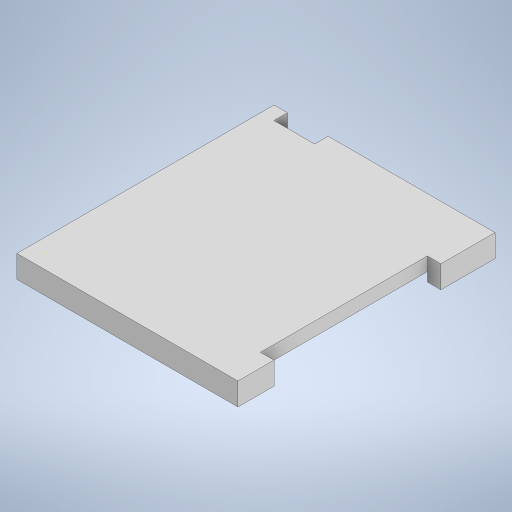
# Autodesk Inventor part: Part9
Saved by Autodesk Inventor 2023 (Build 270158000, 158)
## iProperties
Created: 2024-11-25
Part Number: Part9
Material: Generic
Document SubType Name: Sheet Metal
Designer: 1ZHUSAM
Density: 1 g/cm^3
Sheet Metal Rule: Default_mm
Appearance: Default
Author: 1ZHUSAM
Autodesk Inventor part; units mm, degrees
ref_plane "YZ Plane" through (0, 0, 0) normal (1, 0, 0) x (0, 1, 0)
ref_plane "XZ Plane" through (0, 0, 0) normal (0, 1, 0) x (-1, 0, 0)
ref_plane "XY Plane" through (0, 0, 0) normal (0, 0, 1) x (1, 0, 0)
sketch "Sketch1" plane through (0, 0, 0) normal (0, 1, 0) x (-1, 0, 0)
  line L0 (0, 0) -> (-43, 0)
  line L1 (-43, 0) -> (-43, -51)
  line L2 (-43, -51) -> (0, -51)
  line L3 (0, -51) -> (0, 0)
  line L4 (-43, -51) -> (-46, -51)
  line L5 (-46, -51) -> (-46, -42)
  line L6 (-46, -42) -> (-43, -42)
  line L7 (-43, 0) -> (-46, 0)
  line L8 (-46, 0) -> (-46, -5)
  line L9 (-46, -5) -> (-43, -5)
  line L10 (-43, 0) -> (-46, 0)
  line L11 (-46, 0) -> (-46, 3)
  line L12 (-46, 3) -> (0, 3)
  line L13 (0, 3) -> (0, 0)
  line L14 (0, 3) -> (3, 3)
  line L15 (3, 3) -> (3, -51)
  line L16 (3, -51) -> (0, -51)
  line L17 (3, -51) -> (3, -54)
  line L18 (3, -54) -> (0, -54)
  line L19 (0, -54) -> (0, -51)
  line L20 (-43, -51) -> (-43, -54)
  line L21 (-43, -54) -> (-9, -54)
  line L22 (-9, -54) -> (-9, -51)
  line L23 (-43, -54) -> (-46, -54)
  line L24 (-46, -54) -> (-46, -51)
  dimension "d0" = 43
  dimension "d1" = 51
  dimension "d2" = 3
  dimension "d3" = 9
  dimension "d4" = 3
  dimension "d5" = 5
  dimension "d6" = 3
  dimension "d7" = 3
  dimension "d8" = 3
  dimension "d9" = 3
  dimension "d10" = 3
  dimension "d11" = 34
  constraints: 50 end point, 12 perpendicular, 7 point on line, 4 horizontal, 3 parallel, 2 vertical
  measures "d0" distance of L2.end L1.end
  measures "d1" distance of L1.end L0.end
  measures "d2" distance of L1.end L4.end
  measures "d3" distance of L4.end L5.end
  measures "d4" distance of L0.end L7.end
  measures "d5" distance of L7.end L8.end
  measures "d6" distance of L7.end L11.end
  measures "d7" distance of L12.end L14.end
  measures "d8" distance of L15.end L17.end
  measures "d9" distance of L17.end L18.end
  measures "d10" distance of L1.end L20.end
  measures "d11" distance of L20.end L21.end
sketch "Sketch2" plane through (0, 0, 0) normal (0, 1, 0) x (-1, 0, 0)
  point P0 (0, 0)
extrude "Extrusion1" add sketch "Sketch1" along normal blind 5 contours L13 L14 L15 L16 L3 | L0 L7 L11 L12 L13 | L1 L9 L8 L7 | L16 L17 L18 L19 | L22 L21 L20 L2 | L1 L4 L5 L6 | L20 L23 L24 L4
sketch "Sketch3" plane through (0, 5, 0) normal (0, 1, 0) x (1, 0, 0)
  line L0 (43, 0) -> (0, 0) projected
  line L1 (43, 51) -> (43, 42) projected
  line L2 (0, 0) -> (43, 0)
  line L3 (43, 0) -> (43, 51)
  line L4 (43, 51) -> (0, 51)
  line L5 (0, 51) -> (0, 0)
  constraints: 8 end point, 2 parallel, 1 horizontal, 1 perpendicular
extrude "Extrusion2" add sketch "Sketch3" against normal blind 3
sketch "Sketch4" plane through (0, 5, 0) normal (0, 1, 0) x (1, 0, 0)
  point P0 (0, 0)
equation "\"BendRadius\" = Thickness"
equation "\"BendReliefWidth\" = Thickness"
equation "\"BendReliefDepth\" = 0.5 * Thickness"
equation "\"CornerReliefSize\" = 4 * Thickness"
equation "\"MinimumRemnant\" = 2 * Thickness"
equation "\"TransitionRadius\" = BendRadius"
equation "\"JacobiRadiusSize\" = BendRadius"
equation "\"GapSize\" = Thickness"
equation "\"Thickness\" = 0.5"
body "Solid1"
